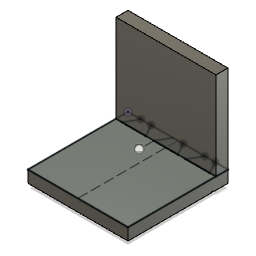
dovetail v1 (Autodesk Fusion 360 design; units mm, degrees)
Autodesk Fusion 360 part; units mm, degrees
sketch "Sketch1" plane through (0, 0, 0) normal (0, 1, 0) x (1, 0, 0)
  line L0 (0, 0) -> (25, 0)
  line L1 (25, 0) -> (25, -25)
  line L2 (25, -25) -> (0, -25)
  line L3 (0, -25) -> (0, 0)
  line L4 (0, -3) -> (25, -3) construction
  line L5 (12.5, 0) -> (12.5, -25) construction
  line L6 (11.2321, 0) -> (9.5, -3)
  line L7 (9.5, -3) -> (9.5, -6.7113) construction
  line L8 (13.7679, 0) -> (15.5, -3)
  line L9 (9.5, -3) -> (15.5, -3)
  line L10 (3.2321, 0) -> (1.5, -3)
  line L11 (5.7679, 0) -> (7.5, -3)
  line L12 (1.5, -3) -> (7.5, -3)
  line L13 (19.2321, 0) -> (17.5, -3)
  line L14 (21.7679, 0) -> (23.5, -3)
  line L15 (17.5, -3) -> (23.5, -3)
  line L16 (0, -3) -> (25, -3)
  dimension "d1" = 25
  dimension "d2" = 25
  dimension "d3" = 3
  dimension "d4" = 150
  dimension "d6" = 3
  dimension "d9" = 8
  dimension "d10" = 0
  constraint horizontal L0
  constraint vertical L1
  constraint horizontal L2
  constraint vertical L3
  constraint coincident L0.start L3.end
  constraint coincident L3 L4.start
  constraint coincident L1 L4.end
  constraint perpendicular L1 L4
  constraint midpoint L0 L5.start
  constraint midpoint L2 L5.end
  constraint coincident L0 L6.start
  constraint coincident L4 L6.end
  constraint perpendicular L4 L7
  constraint symmetric L5 L6.start L8.start
  constraint symmetric L5 L6.end L8.end
  measures "d1" distance of L0.start L0.end
  measures "d2" distance of L0.start L2.end
  measures "d3" distance of L0 L4
  measures "d4" angle of L5 L6
  measures "d6" distance of L5 L7
extrude "Extrude1" add sketch "Sketch1" against normal blind 3 contours L0 L3 L10 L16 | L1 L2 L3 L9 L12 L15 L16 | L0 L6 L11 L16 | L0 L8 L13 L16 | L0 L1 L14 L16 makes body 1
extrude "Extrude2" add sketch "Sketch1" against normal blind 4 separate body contours L0 L10 L11 L12 L16 | L0 L6 L8 L9 L16 | L0 L13 L14 L15 L16 makes body 2 at (3.5, -1.3333, 3) makes body 3 at (11.5, -1.3333, 3) makes body 4 at (19.5, -1.3333, 3)
extrude "Extrude3" add sketch "Sketch1" along normal blind 22 contours L0 L3 L10 L16 | L0 L10 L11 L12 L16 | L0 L6 L11 L16 | L0 L6 L8 L9 L16 | L0 L8 L13 L16 | L0 L1 L14 L16 | L0 L13 L14 L15 L16 bodies 2 3 4
move_face "OffsetFaces1" offset -0.1 9 faces at (2.6547, -1, 1) (10.6547, -1, 1) (18.6547, -1, 1) (5.5, -2, 3) (11.5, -1, 3) (19.5, -1, 3) (22.3453, -1, 1) (14.3453, -1, 1) (6.3453, -1, 1) on bodies 1
chamfer "Chamfer1" distance 1 angle 45 9 edges at (2.2217, -3, 1.55) (4.5, -3, 3.1) (6.7783, -3, 1.55) (10.2217, -3, 1.55) (12.5, -3, 3.1) (14.7783, -3, 1.55) (18.2217, -3, 1.55) (20.5, -3, 3.1) (22.7783, -3, 1.55) on bodies 1
fillet "Fillet1" radius 0.7 6 edges at (1.5, -2, 3) (7.5, -2, 3) (9.5, -2, 3) (15.5, -2, 3) (17.5, -2, 3) (23.5, -2, 3) on bodies 2
named bodies: "dovetail holes", "dovetail pins"
